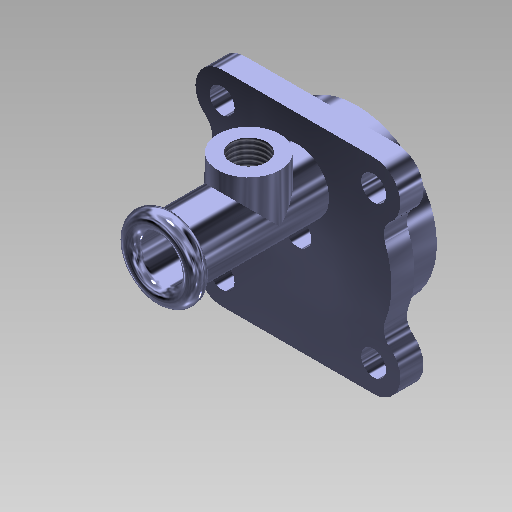
# Autodesk Inventor part: cover
Saved by Autodesk Inventor 2018.1 (Build 221171000, 171)
## iProperties
Created: 2013-08-27
Part Number: cover
Material: Generic
Document SubType Name: Modeling
Designer: Konstantin
Density: 1 g/cm^3
Appearance: Default
Mass: 2.34891 g
Surface Area: 23.2478 cm^2
Volume: 2.34891 cm^3
Author: Konstantin
Autodesk Inventor part; units mm, degrees
ref_plane "XY Plane" through (0, 0, 0) normal (0, 0, 1) x (1, 0, 0)
sketch "Sketch1" plane through (0, 0, 0) normal (0, 0, 1) x (1, 0, 0)
  circle A0 centre (17, 3) radius 1.4
  circle A1 centre (0, 20) radius 1.4
  circle A2 centre (17, 20) radius 1.4
  circle A3 centre (0, 3) radius 1.4
  arc A4 (-1.2644, 15.3609) -> (-1.2644, 7.6391) centre (8.5, 11.5) ccw
  arc A5 (-1.8746, 5.3422) -> (-1.2644, 7.6391) centre (-3.1243, 6.9037) ccw
  arc A6 (-1.8746, 5.3422) -> (0, 0) centre (0, 3) ccw
  line L0 (0, 0) -> (17, 0)
  arc A7 (17, 0) -> (18.8746, 5.3422) centre (17, 3) ccw
  arc A8 (18.2644, 7.6391) -> (18.8746, 5.3422) centre (20.1243, 6.9037) ccw
  arc A9 (18.2644, 7.6391) -> (18.2644, 15.3609) centre (8.5, 11.5) ccw
  arc A10 (18.8746, 17.6578) -> (18.2644, 15.3609) centre (20.1243, 16.0963) ccw
  arc A11 (18.8746, 17.6578) -> (17, 23) centre (17, 20) ccw
  line L1 (17, 23) -> (0, 23)
  arc A12 (0, 23) -> (-1.8746, 17.6578) centre (0, 20) ccw
  arc A13 (-1.2644, 15.3609) -> (-1.8746, 17.6578) centre (-3.1243, 16.0963) ccw
  constraints: 20 point on circle, 14 centre point, 4 end point, 2 horizontal, 14 other
extrude "Extrusion1" add sketch "Sketch1" along normal blind 2.6
sketch "Sketch2" plane through (0, 0, 0) normal (0, 0, -1) x (-1, 0, 0)
  circle A0 centre (-8.5, 11.5) radius 9
  constraints: 1 centre point, 1 other
extrude "Extrusion2" add sketch "Sketch2" along normal blind 4
sketch "Sketch3" plane through (8.5, 11.5, -4) normal (0, 0, -1) x (-1, 0, 0)
  arc A0 (0, 7.5) -> (-5.3033, 5.3033) centre (0, 0) ccw
  arc A1 (0, 2.5) -> (0, 7.5) centre (0, 5) ccw
  arc A2 (0, 2.5) -> (-1.7678, 1.7678) centre (0, 0) ccw
  arc A3 (-5.3033, 5.3033) -> (-1.7678, 1.7678) centre (-3.5355, 3.5355) ccw
  constraints: 8 point on circle, 4 centre point, 1 coincident, 1 equal radius, 3 other
extrude "Extrusion3" cut sketch "Sketch3" against normal blind 4
sketch "Sketch4" plane through (0, 0, 2.6) normal (0, 0, 1) x (1, 0, 0)
  circle A0 centre (8.5, 16.5) radius 3.5
  constraints: 1 centre point, 1 other
extrude "Extrusion4" add sketch "Sketch4" along normal blind 15
ref_plane "Work Plane1" through (8.5, 0, 0) normal (1, 0, 0) x (0, 1, 0)
sketch "Sketch6" plane through (8.5, 0, 0) normal (1, 0, 0) x (0, 1, 0)
  circle A0 centre (20, 17.6) radius 1
  line L0 (16.5, 17.6) -> (16.5, 21.4909) construction
  constraints: 2 end point, 1 centre point, 1 vertical, 1 other
revolve "Revolution1" add sketch "Sketch6" angle 360 about axis through (8.5, 16.5, 17.6) along (0, 0, 1)
ref_plane "Work Plane2" through (0, 20, 0) normal (0, 1, 0) x (-1, 0, 0)
sketch "Sketch7" plane through (0, 20, 0) normal (0, 1, 0) x (-1, 0, 0)
  circle A0 centre (-8.5, 8.1) radius 3.5
  constraints: 1 centre point, 1 other
extrude "Extrusion6" add sketch "Sketch7" along normal blind 2 and the other way blind 3.5
sketch "Sketch8" plane through (8.5, 16.5, 17.6) normal (0, 0, 1) x (1, 0, 0)
  circle A0 centre (0, 0) radius 2.5 projected
extrude "Extrusion8" cut sketch "Sketch8" against normal blind 20
sketch "Sketch9" plane through (8.5, 22, 8.1) normal (0, 1, 0) x (1, 0, 0)
  circle A0 centre (0, 0) radius 2
  constraints: 1 centre point, 1 other
extrude "Extrusion9" cut sketch "Sketch9" against normal blind 5
thread "Thread1" size "M4x0.5" class "6H" standard "ISO Metric profile" full length
sketch "Sketch10" plane through (0, 0, 2.6) normal (0, 0, 1) x (1, 0, 0)
  circle A0 centre (8.5, 11.5) radius 1.5
  constraints: 1 centre point, 1 other
extrude "Extrusion10" cut sketch "Sketch10" against normal blind 10
body "Solid1"
